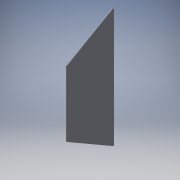
# Autodesk Inventor part: Part7
Saved by Autodesk Inventor 2016 (Build 200138000, 138)
## iProperties
Created: 2016-09-04
Part Number: Part7
Material: Generic
Document SubType Name: Modeling
Designer: gus
Density: 1 g/cm^3
Appearance: Default
Author: gus
Autodesk Inventor part; units mm, degrees
ref_plane "YZ Plane" through (0, 0, 0) normal (1, 0, 0) x (0, 1, 0)
ref_plane "XZ Plane" through (0, 0, 0) normal (0, 1, 0) x (-1, 0, 0)
ref_plane "XY Plane" through (0, 0, 0) normal (0, 0, 1) x (1, 0, 0)
sketch "Sketch1" plane through (0, 0, 0) normal (0, 0, 1) x (1, 0, 0)
  line L0 (0, 0) -> (-3.175, 0)
  line L1 (-3.175, 0) -> (-3.175, -384.175)
  line L2 (-3.175, -384.175) -> (0, -384.175)
  line L3 (0, -384.175) -> (0, 0)
  dimension "d0" = 384.175
  dimension "d1" = 3.175
  constraints: 8 end point, 2 parallel, 1 horizontal, 1 perpendicular
  measures "d0" distance of L2.end L0.start
  measures "d1" distance between parallel lines of L3 L1
extrude "Extrusion1" add sketch "Sketch1" along normal blind 152.4
chamfer "Chamfer1" distance 85.725 angle 60 1 edges at (-1.5875, -384.175, 152.4) measured on face at (-1.0583, -256.1167, 152.4)
chamfer "Chamfer2" distance 85.725 angle 60 1 edges at (-1.5875, 0, 152.4) measured on face at (-1.0583, -198.9667, 152.4)
body "Solid1"
